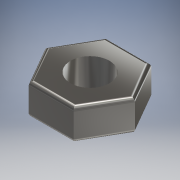
# Autodesk Inventor part: m2 nut
Saved by Autodesk Inventor 2017 (Build 210142000, 142)
## iProperties
Created: 2019-12-06
Part Number: m2 nut
Material: Generic
Document SubType Name: Modeling
Designer: User
Density: 1 g/cm^3
Appearance: Default
Author: User
Autodesk Inventor part; units mm, degrees
ref_plane "YZ Plane" through (0, 0, 0) normal (1, 0, 0) x (0, 1, 0)
ref_plane "XZ Plane" through (0, 0, 0) normal (0, 1, 0) x (-1, 0, 0)
ref_plane "XY Plane" through (0, 0, 0) normal (0, 0, 1) x (1, 0, 0)
sketch "Sketch1" plane through (0, 0, 0) normal (0, 0, 1) x (1, 0, 0)
  circle A0 centre (0, 0) radius 1
  line L0 (-1.1547, -2) -> (1.1547, -2)
  line L1 (1.1547, 2) -> (-1.1547, 2)
  line L2 (1.1547, 2) -> (2.3094, 0)
  line L3 (2.3094, 0) -> (1.1547, -2)
  line L4 (-1.1547, 2) -> (-2.3094, 0)
  line L5 (-2.3094, 0) -> (-1.1547, -2)
  dimension "d0" = 2
  dimension "d5" = 120
  constraints: 12 end point, 1 centre point, 1 coincident, 1 horizontal, 1 parallel
  measures "d0" diameter of A0
  measures "d5" angle of L2 L3
extrude "Extrusion1" add sketch "Sketch1" along normal blind 1.6
fillet "Fillet1" radius 0.2 12 edges at (0, -2, 1.6) (1.7321, -1, 1.6) (1.7321, 1, 1.6) (0, 2, 1.6) (-1.7321, 1, 1.6) (-1.7321, -1, 1.6) (0, 2, 0) (-1.7321, 1, 0) (-1.7321, -1, 0) (0, -2, 0) (1.7321, -1, 0) (1.7321, 1, 0)
body "Solid1"
